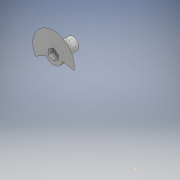
# Autodesk Inventor part: nutholderv2
Saved by Autodesk Inventor 2017 (Build 210142000, 142)
## iProperties
Created: 2017-12-20
Part Number: nutholderv2
Material: Generic
Document SubType Name: Modeling
Designer: will
Density: 1 g/cm^3
Appearance: Default
Author: will
Autodesk Inventor part; units mm, degrees
ref_plane "YZ Plane" through (0, 0, 0) normal (1, 0, 0) x (0, 1, 0)
ref_plane "XZ Plane" through (0, 0, 0) normal (0, 1, 0) x (-1, 0, 0)
ref_plane "XY Plane" through (0, 0, 0) normal (0, 0, 1) x (1, 0, 0)
sketch "Sketch1" plane through (0, 0, 0) normal (0, 1, 0) x (-1, 0, 0)
  line L0 (62.4858, 49.9157) -> (58.4858, 52.2251)
  line L1 (58.4858, 52.2251) -> (58.4858, 56.8439)
  line L2 (58.4858, 56.8439) -> (62.4858, 59.1533)
  line L3 (62.4858, 59.1533) -> (66.4858, 56.8439)
  line L4 (66.4858, 56.8439) -> (66.4858, 52.2251)
  line L5 (66.4858, 52.2251) -> (62.4858, 49.9157)
  line L6 (54.9858, 54.5345) -> (62.4858, 54.5345) construction
  line L7 (62.4858, 54.5345) -> (69.9858, 54.5345) construction
  circle A0 centre (62.4858, 54.5345) radius 7.5
  point P0 (0, 0)
  dimension "d2" = 8
  constraints: 16 end point, 1 centre point, 1 coincident, 1 collinear, 1 horizontal, 1 vertical, 13 other
  measures "d2" distance between parallel lines of L2 L5
extrude "Extrusion1" add sketch "Sketch1" along normal blind 6.25
sketch "Sketch2" plane through (0, 6.25, 0) normal (0, 1, 0) x (1, 0, 0)
  line L0 (-62.4858, -59.1533) -> (-66.4858, -56.8439) projected
  line L1 (-66.4858, -56.8439) -> (-66.4858, -52.2251) projected
  line L2 (-66.4858, -52.2251) -> (-62.4858, -49.9157) projected
  line L3 (-62.4858, -49.9157) -> (-58.4858, -52.2251) projected
  line L4 (-58.4858, -56.8439) -> (-62.4858, -59.1533) projected
  line L5 (-58.4858, -52.2251) -> (-58.4858, -56.8439) projected
  circle A0 centre (-62.4858, -54.5345) radius 2.75
  line L6 (-66.4858, -54.5345) -> (-62.4858, -54.5345) construction
  line L7 (-62.4858, -54.5345) -> (-60.4858, -51.0704) construction
  line L8 (-62.4858, -54.5345) -> (-60.4858, -57.9986) construction
  point P0 (0, 0)
  dimension "d5" = 5.5
  constraints: 6 end point, 3 midpoint, 2 equal length, 1 centre point
  measures "d5" diameter of A0
extrude "Extrusion2" add sketch "Sketch2" against normal blind 2.25
sketch "Sketch3" plane through (-69.9858, 0, 62.0345) normal (0, 0, 1) x (1, 0, 0)
  line L0 (0, 0) -> (15, 0) projected
  line L1 (15, 0) -> (15, 6.25) projected
  line L2 (0, 6.25) -> (15, 6.25) projected
  line L3 (0, 0) -> (0, 6.25) projected
  point P0 (69.9858, 0)
extrude "Extrusion3" [suppressed]
sketch "Sketch4" plane through (0, 6.25, 0) normal (0, 1, 0) x (1, 0, 0)
  point P0 (0, 0)
sketch "Sketch5" plane through (0, 6.25, 0) normal (0, 1, 0) x (1, 0, 0)
  circle A0 centre (-62.4858, -54.5345) radius 2.75 projected
  circle A1 centre (-62.4858, -54.5345) radius 5.0287
  point P0 (0, 0)
  constraints: 1 centre point, 1 coincident
extrude "Extrusion4" add sketch "Sketch5" along normal blind 10
ref_plane "Work Plane1" through (-64.4858, 0, 53.3798) normal (-0.5, 0, 0.8660254) x (0.8660254, 0, 0.5)
sketch "Sketch8" plane through (-64.4858, 0, 53.3798) normal (-0.5, 0, 0.8660254) x (0.8660254, 0, 0.5)
  line L0 (-5.1906, 6.1827) -> (-15.1311, 0)
  line L1 (-15.1311, 0) -> (-5.1906, 0)
  line L2 (-5.1906, 0) -> (-5.1906, 6.1827)
  line L3 (-5.1906, 0) -> (-5.1906, 6.25) projected
  line L4 (7.3381, 16.25) -> (-2.7193, 16.25) projected
  line L5 (2.3094, 16.25) -> (2.3094, 0)
  line L6 (-5.1906, 0) -> (9.8094, 0) projected
  point P0 (29.1564, 0)
  constraints: 8 end point, 2 midpoint, 1 collinear
revolve "Revolution1" add sketch "Sketch8" angle 220 about axis through (-62.4858, 16.25, 54.5345) along (0, 1, 0)
body "Solid1"
